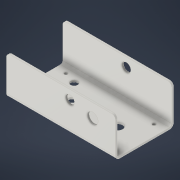
# Autodesk Inventor part: dekiel
Saved by Autodesk Inventor 2022 (Build 260153000, 153)
## iProperties
Created: 2021-03-29
Part Number: dekiel
Material: Stal
Document SubType Name: Konstrukcja blachowa
Designer: Karol
Density: 7.85 g/cm^3
Sheet Metal Rule: Domyślny_mm
Appearance: Stal
Flat Pattern Width: 12 cm
Flat Pattern Length: 14.2619 cm
Flat Pattern Area: 171.142 cm^2
Sheet Metal Width: 120,000 mm
Sheet Metal Length: 142,619 mm
Sheet Metal Area: 17114,230 mm^2
Author: Karol
Autodesk Inventor part; units mm, degrees
ref_plane "YZ Plane" through (0, 0, 0) normal (1, 0, 0) x (0, 1, 0)
ref_plane "XZ Plane" through (0, 0, 0) normal (0, 1, 0) x (-1, 0, 0)
ref_plane "XY Plane" through (0, 0, 0) normal (0, 0, 1) x (1, 0, 0)
sketch "Szkic1" plane through (0, 0, 0) normal (0, 1, 0) x (-1, 0, 0)
  line L0 (-60, -30) -> (60, -30)
  line L1 (60, -30) -> (60, 30)
  line L2 (60, 30) -> (-60, 30)
  line L3 (-60, 30) -> (-60, -30)
  line L4 (-60, -30) -> (60, 30) construction
  line L5 (60, -30) -> (-60, 30) construction
  point P0 (0, 0)
  dimension "d0" = 120
  dimension "d1" = 60
  measures "d0" distance of L2.end L1.end
  measures "d1" distance of L0.end L1.end
extrude "Płyta1" add sketch "Szkic1" along normal blind 2
sketch "Szkic2" plane through (60, 2, 30) normal (0, 0, 1) x (1, 0, 0)
  line L0 (-120, 0) -> (0, 0)
  line L1 (0, 0) -> (0, 41)
  line L2 (0, 41) -> (-120, 41)
  line L3 (-120, 41) -> (-120, 0)
  constraints: 6 end point, 1 horizontal, 1 perpendicular, 1 vertical
edge flange "Kołnierz1" height 43 angle 90 thickness 2 bend radius 2.5 thickness toward (0, 0, 1) relief tear relief width 2 relief depth 1 corner gap 2 corner form 0 edges at (0, 2, 30) (0, 2, -30) wall of the first edge with corners at (-60, 2, 30) (60, 2, 30) (60, 43, 30) (-60, 43, 30)
bend "Zagięcie1"
corner "Narożnik1"
sketch "Szkic3" plane through (0, 2, 0) normal (0, 1, 0) x (1, 0, 0)
  circle A0 centre (48.5, 22) radius 1.2295 projected
  circle A1 centre (48.5, -22) radius 1.2295 projected
  circle A2 centre (-48.5, 22) radius 1.2295 projected
  circle A3 centre (-48.5, -22) radius 1.2295 projected
  point P0 (0, 0)
  constraints: 4 coincident
hole "Otwór1" at (48.5, 2, -22) at (48.5, 2, 22) at (-48.5, 2, -22) at (-48.5, 2, 22) direction (0, -1, 0) diameter 3.5 depth 2 tip angle 118 clearance for "Śruba ze łbem płaskim obrobiona" size "M3" standard "ANSI Profil metryczny M"
fillet "Zaokrąglenie1" radius 4 4 edges at (-60, 43, -31) (-60, 43, 31) (60, 43, 31) (60, 43, -31)
sketch "Szkic4" plane through (0, 0, 0) normal (0, -1, 0) x (1, 0, 0)
  circle A0 centre (-20, 0) radius 4
  circle A1 centre (-35, 17.5) radius 4
  circle A2 centre (-35, -17.5) radius 4
  line L0 (-60, -27.5) -> (-60, 27.5) projected
  point P0 (0, 0)
  dimension "d22" = 35
  dimension "d23" = 17.5
  dimension "d24" = 15
  dimension "d25" = 8
  dimension "d26" = 25
  constraints: 3 centre point, 2 equal radius, 1 horizontal alignment, 1 vertical alignment
  measures "d22" distance of A1.centre A2.centre
  measures "d23" vertical distance of point (0, 0) A1.centre
  measures "d24" horizontal distance of A1.centre A0.centre
  measures "d25" diameter of A2
  measures "d26" distance from line of L0 A2.centre
extrude "Wytnij1" cut sketch "Szkic4" against normal blind 2
sketch "Szkic5" plane through (0, 0, 0) normal (0, -1, 0) x (1, 0, 0)
  circle A0 centre (30, 0) radius 6
  line L0 (60, 27.5) -> (60, -27.5) projected
  point P0 (0, 0)
  point P1 (60, 0)
  dimension "d29" = 12
  dimension "d30" = 30
  constraints: 1 centre point, 1 horizontal alignment, 1 midpoint
  measures "d29" diameter of A0
  measures "d30" distance from line of L0 A0.centre
extrude "Wytnij2" cut sketch "Szkic5" against normal blind 2
sketch "Szkic6" plane through (60, 4.5, -32) normal (0, 0, -1) x (-1, 0, 0)
  circle A0 centre (50, 28.5) radius 5
  line L0 (4, 38.5) -> (116, 38.5) projected
  line L1 (0, 0) -> (0, 34.5) projected
  point P0 (60, -4.5)
  dimension "d33" = 10
  dimension "d34" = 10
  dimension "d35" = 50
  constraints: 1 centre point
  measures "d33" diameter of A0
  measures "d34" distance from line of L0 A0.centre
  measures "d35" distance from line of L1 A0.centre
extrude "Wytnij3" cut sketch "Szkic6" against normal through all
sketch "Szkic7" plane through (0, 0, 0) normal (0, -1, 0) x (1, 0, 0)
  circle A0 centre (-37, 0) radius 4
  line L0 (-60, -27.5) -> (-60, 27.5) projected
  point P0 (0, 0)
  point P1 (-60, 0)
  dimension "d38" = 8
  dimension "d39" = 23
  constraints: 1 centre point, 1 horizontal alignment, 1 midpoint
  measures "d38" diameter of A0
  measures "d39" distance from line of L0 A0.centre
extrude "Wytnij4" cut sketch "Szkic7" against normal blind 2
sketch "Szkic8" plane through (-60, 4.5, 32) normal (0, 0, 1) x (1, 0, 0)
  circle A0 centre (95, 23.5) radius 6
  line L0 (120, 34.5) -> (120, 0) projected
  circle A1 centre (70, 28.5) radius 5 projected
  line L1 (4, 38.5) -> (116, 38.5) projected
  point P0 (60, -4.5)
  dimension "d42" = 12
  dimension "d43" = 25
  dimension "d46" = 15
  constraints: 1 centre point
  measures "d42" diameter of A0
  measures "d43" distance from line of L0 A0.centre
  measures "d46" distance from line of A0.centre L1
extrude "Wytnij5" cut sketch "Szkic8" against normal blind 2 contours A0
equation "\"d19\" = Grubość"
equation "\"d23\" = 0.5 * d22"
equation "\"d27\" = Grubość"
equation "\"d31\" = Grubość"
equation "\"d36\" = Grubość"
equation "\"d40\" = Grubość"
equation "\"d44\" = Grubość"
equation "\"d2\" = Grubość"
equation "\"d3\" = SzerokośćGięciaPodcięcia"
equation "\"d4\" = GłębokośćGięciaPodcięcia"
equation "\"d5\" = MinimalnaPozostałość"
equation "\"d6\" = PromieńPrzejścia"
equation "\"d10\" = RozmiarPodcięciaNarożnika"
equation "\"d11\" = Wielk_odstępu"
equation "\"d12\" = Rozmiar_promienia_Jacobiego"
equation "\"PromieńGięcia\" = Grubość"
equation "\"SzerokośćGięciaPodcięcia\" = Grubość"
equation "\"GłębokośćGięciaPodcięcia\" = 0.5 * Grubość"
equation "\"RozmiarPodcięciaNarożnika\" = 4 * Grubość"
equation "\"MinimalnaPozostałość\" = 2 * Grubość"
equation "\"PromieńPrzejścia\" = PromieńGięcia"
equation "\"Rozmiar_promienia_Jacobiego\" = PromieńGięcia"
equation "\"Wielk_odstępu\" = Grubość"
equation "\"Grubość\" = 2"
